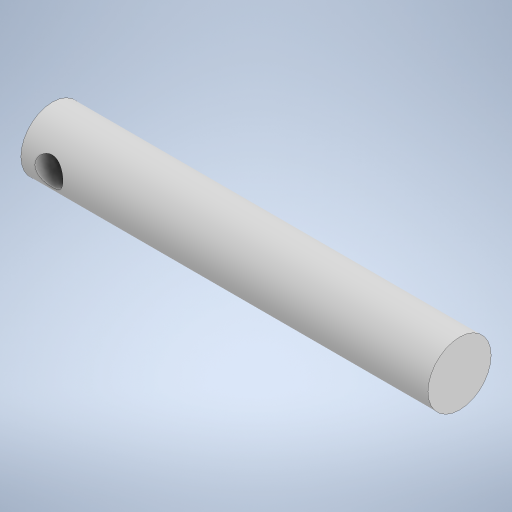
# Autodesk Inventor part: Hudson 1-62B
Saved by Autodesk Inventor 2024.2 (Build 282272000, 272)
## iProperties
Created: 2024-10-07
Part Number: Hudson 1-62B
Material: Genérico
Document SubType Name: Modeling
Designer: Monica Mora
Density: 1 g/cm^3
Appearance: Valor por defecto
Author: Monica Mora
Autodesk Inventor part; units mm, degrees
ref_plane "YZ Plane" through (0, 0, 0) normal (1, 0, 0) x (0, 1, 0)
ref_plane "XZ Plane" through (0, 0, 0) normal (0, 1, 0) x (-1, 0, 0)
ref_plane "XY Plane" through (0, 0, 0) normal (0, 0, 1) x (1, 0, 0)
sketch "Boceto1" plane through (0, 0, 0) normal (0, 0, 1) x (1, 0, 0)
  line L0 (0, 0) -> (-29, 0)
  line L1 (-29, 0) -> (-29, 2.25)
  line L2 (-29, 2.25) -> (0, 2.25)
  line L3 (0, 2.25) -> (0, 0)
  dimension "d0" = 29
  dimension "d1" = 4.5
  constraints: 8 end point, 2 perpendicular, 1 horizontal, 1 vertical
  measures "d0" distance of L0.start L0.end
  measures "d1" diameter of L2 L0
revolve "Revolución1" add sketch "Boceto1" angle 360 about axis through (0, 0, 0) along (-1, 0, 0)
sketch "Boceto2" plane through (0, 0, 0) normal (0, 0, 1) x (1, 0, 0)
  line L0 (0, 2.25) -> (0, -2.25) projected
  line L1 (0, -2.25) -> (-29, -2.25) projected
  line L2 (-29, -2.25) -> (-29, 2.25) projected
  line L3 (-29, 2.25) -> (0, 2.25) projected
  line L4 (-29, 0) -> (0, 0) construction
  line L5 (-27, 2.25) -> (-27, -2.25) construction
  circle A0 centre (-27, 0) radius 1
  dimension "d3" = 2
  dimension "d4" = 2
  constraints: 4 end point, 2 midpoint, 2 point on line, 1 centre point, 1 horizontal, 1 perpendicular
  measures "d3" distance between parallel lines of L2 L5
  measures "d4" diameter of A0
hole "Agujero1" at (-27, 0, 0) direction (0, 0, -1) diameter 2 end through all both
